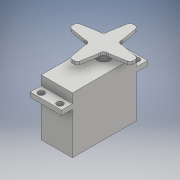
# Autodesk Inventor part: FutabaS3003Rough
Saved by Autodesk Inventor 2018 (Build 220112000, 112)
## iProperties
Created: 2017-07-30
Part Number: FutabaS3003Rough
Material: Generic
Document SubType Name: Modeling
Designer: kurtis
Density: 1 g/cm^3
Appearance: Default
Author: kurtis
Autodesk Inventor part; units mm, degrees
ref_plane "YZ Plane" through (0, 0, 0) normal (1, 0, 0) x (0, 1, 0)
ref_plane "XZ Plane" through (0, 0, 0) normal (0, 1, 0) x (-1, 0, 0)
ref_plane "XY Plane" through (0, 0, 0) normal (0, 0, 1) x (1, 0, 0)
sketch "Sketch1" plane through (0, 0, 0) normal (0, 0, 1) x (1, 0, 0)
  line L0 (0, 0) -> (20, 0)
  line L1 (20, 0) -> (20, 41)
  line L2 (20, 41) -> (0, 41)
  line L3 (0, 41) -> (0, 0)
  dimension "d0" = 20
  dimension "d1" = 41
  constraints: 8 end point, 2 parallel, 1 horizontal, 1 perpendicular
  measures "d0" distance of L2.end L1.end
  measures "d1" distance of L1.end L0.end
extrude "Extrusion1" add sketch "Sketch1" along normal blind 27
sketch "Sketch2" plane through (0, 0, 27) normal (0, 0, 1) x (1, 0, 0)
  line L0 (0, 41) -> (0, 0) construction
  line L1 (20, 0) -> (20, 41) construction
  line L2 (0, 0) -> (20, 41) construction
  line L3 (20, 41) -> (0, 41) construction
  line L4 (0, 41) -> (20, 0) construction
  line L5 (0, -7) -> (20, -7)
  line L6 (20, -7) -> (20, 48)
  line L7 (20, 48) -> (0, 48)
  line L8 (0, 48) -> (0, -7)
  line L9 (0, -7) -> (20, 48) construction
  line L10 (20, -7) -> (0, 48) construction
  line L11 (0, 41) -> (0, 45) construction
  line L12 (0, 45) -> (20, 45) construction
  line L13 (0, 45) -> (4, 45) construction
  circle A0 centre (4, 45) radius 2
  line L14 (20, 45) -> (16, 45) construction
  circle A1 centre (16, 45) radius 2
  line L15 (0, 0) -> (20, 0) construction
  line L16 (0, 0) -> (0, -4) construction
  line L17 (0, -4) -> (4, -4) construction
  line L18 (20, 0) -> (20, -4) construction
  line L19 (20, -4) -> (16, -4) construction
  circle A2 centre (4, -4) radius 2
  circle A3 centre (16, -4) radius 2
  point P0 (10, 20.5)
  dimension "d4" = 20
  dimension "d5" = 55
  dimension "d6" = 4
  dimension "d7" = 4
  dimension "d8" = 4
  dimension "d9" = 4
  dimension "d10" = 4
  dimension "d11" = 4
  dimension "d12" = 4
  dimension "d13" = 4
  dimension "d14" = 4
  dimension "d15" = 4
  dimension "d16" = 4
  constraints: 34 end point, 6 point on line, 5 perpendicular, 4 centre point, 4 coincident, 3 midpoint, 3 parallel, 1 horizontal
  measures "d4" distance of L7.end L6.end
  measures "d5" distance of L6.end L5.end
  measures "d6" distance of L3.end L11.end
  measures "d7" distance of L11.end L13.end
  measures "d8" diameter of A0
  measures "d9" distance of L12.end L14.end
  measures "d10" diameter of A1
  measures "d11" distance of L0.end L16.end
  measures "d12" distance of L16.end L17.end
  measures "d13" distance of L1.start L18.end
  measures "d14" distance of L18.end L19.end
  measures "d15" diameter of A2
  measures "d16" diameter of A3
extrude "Extrusion2" add sketch "Sketch2" along normal blind 3
sketch "Sketch3" plane through (0, 0, 30) normal (0, 0, 1) x (1, 0, 0)
  line L0 (0, 48) -> (0, 41) construction
  line L1 (0, -7) -> (20, -7) construction
  line L2 (0, 48) -> (20, -7) construction
  line L3 (20, 41) -> (20, 48) construction
  line L4 (0, -7) -> (20, 48) construction
  line L5 (0, 0) -> (20, 0)
  line L6 (20, 0) -> (20, 41)
  line L7 (20, 41) -> (0, 41)
  line L8 (0, 41) -> (0, 0)
  line L9 (0, 0) -> (20, 41) construction
  line L10 (20, 0) -> (0, 41) construction
  point P0 (10, 20.5)
  dimension "d19" = 20
  dimension "d20" = 41
  constraints: 16 end point, 3 midpoint, 2 parallel, 1 horizontal, 1 perpendicular
  measures "d19" distance of L7.end L3.start
  measures "d20" distance of L3.start L5.end
extrude "Extrusion3" add sketch "Sketch3" along normal blind 6
sketch "Sketch4" plane through (0, 0, 36) normal (0, 0, 1) x (1, 0, 0)
  line L0 (20, 48) -> (0, 48) construction
  line L1 (10, 48) -> (10, 30) construction
  circle A0 centre (10, 30) radius 4
  point P0 (0, 0)
  dimension "d23" = 18
  dimension "d24" = 8
  constraints: 2 end point, 1 centre point, 1 coincident, 1 midpoint, 1 vertical
  measures "d23" distance of L1.start L1.end
  measures "d24" diameter of A0
extrude "Extrusion4" add sketch "Sketch4" along normal blind 8
sketch "Sketch5" plane through (10, 30, 44) normal (0, 0, 1) x (1, 0, 0)
  line L0 (19.5, -0.7059) -> (19.5, 0.7059)
  line L1 (-19.5, 0.7059) -> (-19.5, -0.7059)
  line L2 (-19.5, -4.5) -> (19.5, 4.5) construction
  line L3 (19.5, -4.5) -> (-19.5, 4.5) construction
  line L4 (-0.7059, 19.5) -> (0.7059, 19.5)
  line L5 (0.7059, -19.5) -> (-0.7059, -19.5)
  line L6 (-4.5, 19.5) -> (4.5, -19.5) construction
  line L7 (4.5, 19.5) -> (-4.5, -19.5) construction
  line L8 (4.5, 7.5) -> (4.5, 6.5)
  line L9 (4.5, -6.5) -> (4.5, -7.5)
  line L10 (-4.5, -7.5) -> (-4.5, -6.5)
  line L11 (-4.5, 6.5) -> (-4.5, 7.5)
  line L12 (-7.5, -4.5) -> (-6.5, -4.5)
  line L13 (6.5, -4.5) -> (7.5, -4.5)
  line L14 (7.5, 4.5) -> (6.5, 4.5)
  line L15 (-6.5, 4.5) -> (-7.5, 4.5)
  arc A0 (-6.5, 4.5) -> (-4.5, 6.5) centre (-6.5, 6.5) ccw
  arc A1 (4.5, 6.5) -> (6.5, 4.5) centre (6.5, 6.5) ccw
  arc A2 (6.5, -4.5) -> (4.5, -6.5) centre (6.5, -6.5) ccw
  arc A3 (-4.5, -6.5) -> (-6.5, -4.5) centre (-6.5, -6.5) ccw
  line L16 (4.5, 7.5) -> (2.6755, 17.8473)
  line L17 (-4.5, 7.5) -> (-2.6755, 17.8473)
  line L18 (7.5, -4.5) -> (17.8473, -2.6755)
  line L19 (7.5, 4.5) -> (17.8473, 2.6755)
  line L20 (-7.5, 4.5) -> (-17.8473, 2.6755)
  line L21 (-7.5, -4.5) -> (-17.8473, -2.6755)
  line L22 (-4.5, -7.5) -> (-2.6755, -17.8473)
  line L23 (4.5, -7.5) -> (2.6755, -17.8473)
  arc A4 (-17.8473, 2.6755) -> (-19.5, 0.7059) centre (-17.5, 0.7059) ccw
  arc A5 (-19.5, -0.7059) -> (-17.8473, -2.6755) centre (-17.5, -0.7059) ccw
  arc A6 (-0.7059, 19.5) -> (-2.6755, 17.8473) centre (-0.7059, 17.5) ccw
  arc A7 (2.6755, 17.8473) -> (0.7059, 19.5) centre (0.7059, 17.5) ccw
  arc A8 (19.5, 0.7059) -> (17.8473, 2.6755) centre (17.5, 0.7059) ccw
  arc A9 (17.8473, -2.6755) -> (19.5, -0.7059) centre (17.5, -0.7059) ccw
  arc A10 (-2.6755, -17.8473) -> (-0.7059, -19.5) centre (-0.7059, -17.5) ccw
  arc A11 (0.7059, -19.5) -> (2.6755, -17.8473) centre (0.7059, -17.5) ccw
  point P0 (-10, -30)
  point P1 (0, 0)
  point P2 (0, 0)
  dimension "d27" = 39
  dimension "d28" = 9
  dimension "d29" = 9
  dimension "d30" = 39
  dimension "d31" = 29.5
  dimension "d32" = 49.5
  dimension "d33" = 2
  dimension "d34" = 12
  dimension "d35" = 10
  dimension "d36" = 12
  dimension "d37" = 10
  dimension "d38" = 12
  dimension "d39" = 10
  dimension "d40" = 12
  dimension "d41" = 10
  dimension "d42" = 12
  dimension "d43" = 10
  dimension "d44" = 12
  dimension "d45" = 10
  dimension "d46" = 12
  dimension "d47" = 10
  dimension "d48" = 12
  dimension "d49" = 10
  dimension "d50" = 2
  dimension "d51" = 2
  constraints: 48 end point, 28 tangent, 24 point on circle, 16 point on line, 12 centre point, 10 parallel, 9 equal radius, 5 midpoint, 4 perpendicular, 3 horizontal
  measures "d27" distance of L3.end L2.end
  measures "d28" distance of L2.end L3.start
  measures "d29" distance of L6.end L7.end
  measures "d30" distance of L7.start L6.end
  measures "d31" distance from line of point (-10, -30) L0
  measures "d32" distance from line of point (-10, -30) L4
  measures "d33" radius of A0
  measures "d34" distance of L8.start L7.start
  measures "d35" angle of L8 L16
  measures "d36" distance of L11.end L6.start
  measures "d37" angle of L11 L17
  measures "d38" distance of L13.end L3.start
  measures "d39" angle of L13 L18
  measures "d40" distance of L14.start L2.end
  measures "d41" angle of L14 L19
  measures "d42" distance of L15.end L3.end
  measures "d43" angle of L15 L20
  measures "d44" distance of L12.start L2.start
  measures "d45" angle of L12 L21
  measures "d46" distance of L10.start L7.end
  measures "d47" angle of L10 L22
  measures "d48" distance of L9.end L6.end
  measures "d49" angle of L9 L23
  measures "d50" radius of A4
  measures "d51" radius of A6
extrude "Extrusion5" add sketch "Sketch5" against normal blind 2
equation "\"d36\" = d34"
equation "\"d37\" = d35"
equation "\"d38\" = d34"
equation "\"d39\" = d35"
equation "\"d40\" = d34"
equation "\"d41\" = d35"
equation "\"d42\" = d34"
equation "\"d43\" = d35"
equation "\"d44\" = d34"
equation "\"d45\" = d35"
equation "\"d46\" = d34"
equation "\"d47\" = d35"
equation "\"d48\" = d34"
equation "\"d49\" = d35"
body "Solid1"
